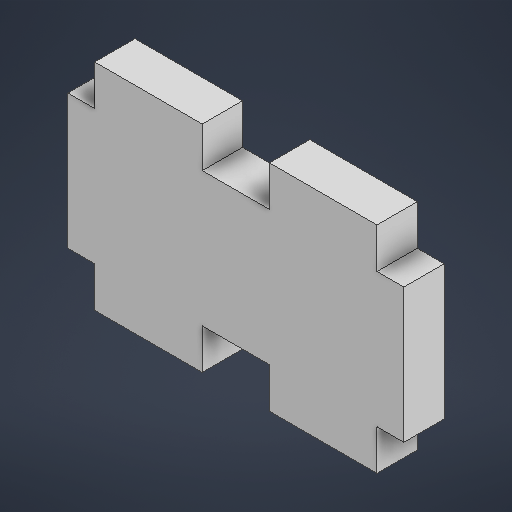
# Autodesk Inventor part: protector hal
Saved by Autodesk Inventor 2026 (Build 300175000, 175)
## iProperties
Created: 2026-05-15
Part Number: protector hal
Material: Generic
Document SubType Name: Modeling
Designer: juana
Density: 1 g/cm^3
Appearance: Default
Author: juana
Autodesk Inventor part; units mm, degrees
ref_plane "YZ Plane" through (0, 0, 0) normal (1, 0, 0) x (0, 1, 0)
ref_plane "XZ Plane" through (0, 0, 0) normal (0, 1, 0) x (-1, 0, 0)
ref_plane "XY Plane" through (0, 0, 0) normal (0, 0, 1) x (1, 0, 0)
sketch "Sketch1" plane through (0, 0, 0) normal (0, 0, 1) x (1, 0, 0)
  line L0 (0, 0) -> (25, 0)
  line L1 (25, 0) -> (25, 10)
  line L2 (25, 10) -> (0, 10)
  line L3 (0, 10) -> (0, 0)
  line L4 (2, 0) -> (10, 0)
  line L5 (10, 0) -> (10, -3)
  line L6 (10, -3) -> (2, -3)
  line L7 (2, -3) -> (2, 0)
  line L8 (12.5, 0) -> (12.5, 10) construction
  line L9 (0, 5) -> (25, 5) construction
  line L10 (15, 0) -> (15, -3)
  line L11 (15, -3) -> (23, -3)
  line L12 (23, -3) -> (23, 0)
  line L13 (10, 10) -> (10, 13)
  line L14 (10, 13) -> (2, 13)
  line L15 (2, 13) -> (2, 10)
  line L16 (15, 13) -> (23, 13)
  line L17 (15, 10) -> (15, 13)
  line L18 (23, 13) -> (23, 10)
  point P0 (23, 0)
  point P1 (15, 0)
  point P2 (10, 0)
  point P3 (15, 10)
  point P4 (23, 10)
  dimension "d0" = 25
  dimension "d1" = 10
  dimension "d5" = 3
  dimension "d6" = 2
  dimension "d7" = 8
  constraints: 38 end point, 12 symmetric about line, 4 midpoint, 4 parallel, 2 horizontal, 2 perpendicular, 1 point on line
  measures "d0" distance of L1.end L2.end
  measures "d1" distance of L0.end L1.end
  measures "d5" distance of L4.end L5.end
  measures "d6" distance between parallel lines of L3 L7
  measures "d7" distance of L5.end L6.end
extrude "Extrusion1" add sketch "Sketch1" along normal blind 3
body "Solid1"
